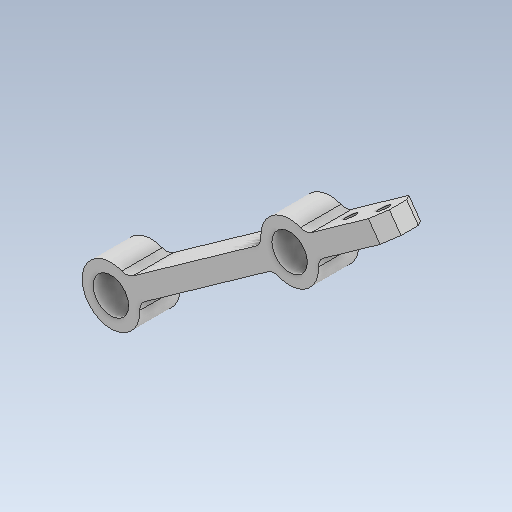
# Autodesk Inventor part: leg_link_1
Saved by Autodesk Inventor 2023 (Build 270158000, 158)
## iProperties
Created: 2020-12-12
Part Number: leg_link_1
Material: Generic
Document SubType Name: Modeling
Designer: Shuang Peng
Density: 1 g/cm^3
Appearance: Default
Author: Shuang Peng
Autodesk Inventor part; units mm, degrees
ref_plane "YZ Plane" through (0, 0, 0) normal (1, 0, 0) x (0, 1, 0)
ref_plane "XZ Plane" through (0, 0, 0) normal (0, 1, 0) x (-1, 0, 0)
ref_plane "XY Plane" through (0, 0, 0) normal (0, 0, 1) x (1, 0, 0)
sketch "Sketch1" plane through (0, 0, 0) normal (0, 0, 1) x (1, 0, 0)
  line L0 (-49.634624, 71.104228) -> (-18.657482, 93.113696)
  circle A0 centre (-49.634624, 71.104228) radius 5
  circle A1 centre (-18.657482, 93.113696) radius 5
  circle A2 centre (-49.634624, 71.104228) radius 3.075
  circle A3 centre (-18.657482, 93.113696) radius 3.075
  line L1 (-49.634624, 71.104228) -> (-18.657482, 93.113696) construction
  line L2 (-48.62103, 69.677649) -> (-17.643888, 91.687117)
  line L3 (-19.671076, 94.540275) -> (-50.648218, 72.530807)
  arc A4 (-50.648218, 72.530807) -> (-48.62103, 69.677649) centre (-49.634624, 71.104228) ccw
  arc A5 (-17.643888, 91.687117) -> (-19.671076, 94.540275) centre (-18.657482, 93.113696) ccw
  line L4 (-18.657482, 93.113696) -> (-2.353723, 104.697626) construction
  line L5 (-17.643888, 91.687117) -> (-1.340129, 103.271047)
  line L6 (-3.367317, 106.124205) -> (-19.671076, 94.540275)
  arc A6 (-19.671076, 94.540275) -> (-17.643888, 91.687117) centre (-18.657482, 93.113696) ccw
  arc A7 (-1.340129, 103.271047) -> (-3.367317, 106.124205) centre (-2.353723, 104.697626) ccw
  line L7 (-2.353723, 104.697626) -> (-3.367317, 106.124205)
  line L8 (-2.353723, 104.697626) -> (-1.340129, 103.271047)
  point P0 (0, 0)
  point P1 (-34.146053, 82.108962)
  point P2 (-10.505602, 98.905661)
  point P3 (-44.802894, 72.39046)
  point P4 (-21.462023, 88.974306)
  point P5 (-13.825752, 94.399928)
  point P6 (-15.85294, 97.253085)
  point P7 (-23.489211, 91.827464)
  point P8 (-46.830082, 75.243618)
  dimension "d0" = 10
  dimension "d1" = 10
  dimension "d2" = 6.15
  dimension "d3" = 6.15
  dimension "d4" = 3.5
  dimension "d5" = 20
  dimension "d6" = 3.5
  constraints: 22 end point, 8 centre point, 8 point on circle, 8 tangent, 4 coincident, 2 collinear, 2 midpoint, 2 parallel
  measures "d0" diameter of A0
  measures "d1" diameter of A1
  measures "d2" diameter of A2
  measures "d3" diameter of A3
  measures "d4" diameter of A5
  measures "d5" distance of L1.end L4.end
  measures "d6" diameter of A7
sketch "Sketch1 outline for Extrusion1" plane through (0, 0, 0) normal (0, 0, 1) x (1, 0, 0)
  line L0 (-44.802894, 72.39046) -> (-21.462023, 88.974306)
  arc A0 (-46.830082, 75.243618) -> (-44.802894, 72.39046) centre (-49.634624, 71.104228) ccw
  arc A1 (-21.462023, 88.974306) -> (-13.825752, 94.399928) centre (-18.657482, 93.113696) ccw
  line L1 (-23.489211, 91.827464) -> (-46.830082, 75.243618)
  line L2 (-13.825752, 94.399928) -> (-1.340129, 103.271047)
  arc A2 (-15.85294, 97.253085) -> (-23.489211, 91.827464) centre (-18.657482, 93.113696) ccw
  line L3 (-1.340129, 103.271047) -> (-2.353723, 104.697626)
  line L4 (-3.367317, 106.124205) -> (-15.85294, 97.253085)
  line L5 (-2.353723, 104.697626) -> (-3.367317, 106.124205)
  circle A3 centre (-49.634624, 71.104228) radius 3.075
  circle A4 centre (-18.657482, 93.113696) radius 3.075
extrude "Extrusion1" add sketch "Sketch1 outline for Extrusion1" along normal mid plane 7
sketch "Sketch2" plane through (-1.340129, 103.271047, -3.5) normal (0.5791965, -0.8151879, 0) x (0.8151879, 0.5791965, 0)
  line L0 (0, 0) -> (0, 7)
  line L1 (-15.316252, 7) -> (0, 7)
  line L2 (-15.316252, 0) -> (-15.316252, 7)
  line L3 (0, 0) -> (-15.316252, 0)
  line L4 (0, 0) -> (0, 7)
  line L5 (0, 3.5) -> (-8, 3.5)
  line L6 (-8, 3.5) -> (-3, 3.5)
  circle A0 centre (-3, 3.5) radius 1
  line L7 (-8, 3.5) -> (-10, 3.5)
  circle A1 centre (-10, 3.5) radius 1
  point P0 (-58.721774, 3.5)
  dimension "d9" = 8
  dimension "d10" = 5
  dimension "d11" = 2
  dimension "d12" = 2
  dimension "d13" = 2
  constraints: 6 end point, 2 centre point, 2 coincident, 2 horizontal, 1 midpoint, 1 point on line
  measures "d9" distance of L5.start L5.end
  measures "d10" distance of L5.end L6.end
  measures "d11" diameter of A0
  measures "d12" distance of L5.end L7.end
  measures "d13" diameter of A1
sketch "Sketch2 outline for Extrusion2" plane through (-1.340129, 103.271047, -3.5) normal (0.5791965, -0.8151879, 0) x (0.8151879, 0.5791965, 0)
  circle A0 centre (-3, 3.5) radius 1
  circle A1 centre (-10, 3.5) radius 1
extrude "Extrusion2" cut sketch "Sketch2 outline for Extrusion2" against normal blind 5
fillet "Fillet1" radius 2 6 edges at (-46.8301, 75.2436, 0) (-44.8029, 72.3905, 0) (-21.462, 88.9743, 0) (-13.8258, 94.3999, 0) (-15.8529, 97.2531, 0) (-23.4892, 91.8275, 0)
chamfer "Chamfer1" distance 2 angle 45 2 edges at (-2.3537, 104.6976, 3.5) (-2.3537, 104.6976, -3.5)
body "Solid1"
